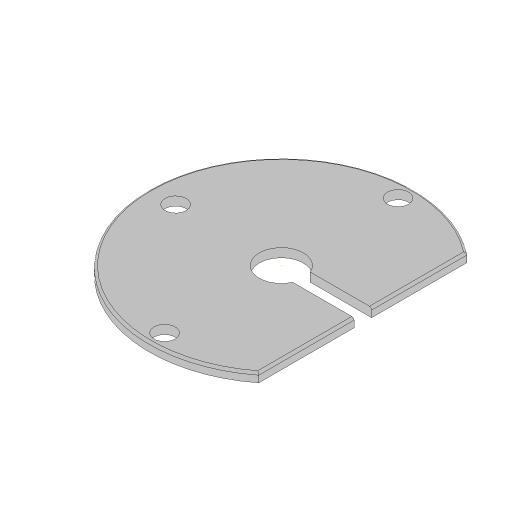
# Autodesk Inventor part: webcam_holder_center_part2
Saved by Autodesk Inventor 2023 (Build 270158000, 158)
## iProperties
Created: 2024-01-25
Part Number: webcam_holder_center_part2
Material: Generic
Document SubType Name: Modeling
Designer: qg3473
Density: 1 g/cm^3
Appearance: Default
Author: qg3473
Autodesk Inventor part; units mm, degrees
ref_plane "YZ Plane" through (0, 0, 0) normal (1, 0, 0) x (0, 1, 0)
ref_plane "XZ Plane" through (0, 0, 0) normal (0, 1, 0) x (-1, 0, 0)
ref_plane "XY Plane" through (0, 0, 0) normal (0, 0, 1) x (1, 0, 0)
sketch "Sketch1" plane through (0, 0, 0) normal (0, 1, 0) x (-1, 0, 0)
  arc A0 (-18.5, -23.6167) -> (-18.5, 23.6167) centre (0, 0) ccw
  line L0 (30, 0) -> (24, 0)
  circle A1 centre (24, 0) radius 2.4
  line L1 (0, 30) -> (0, 26.5)
  line L2 (0, -30) -> (0, -26.5)
  circle A2 centre (0, 26.5) radius 2.4
  circle A3 centre (0, -26.5) radius 2.4
  circle A4 centre (0, 0) radius 5
  line L3 (-30, 0) -> (-18.5, 0)
  line L4 (-18.5, 23.6167) -> (-18.5, -23.6167)
  dimension "d0" = 60
  dimension "d1" = 6
  dimension "d2" = 4.8
  dimension "d3" = 3.5
  dimension "d4" = 3.5
  dimension "d5" = 4.8
  dimension "d6" = 4.8
  dimension "d7" = 10
  dimension "d8" = 11.5
  constraints: 10 end point, 5 centre point, 5 coincident, 5 point on circle, 3 vertical, 2 horizontal
  measures "d0" diameter of A0
  measures "d1" distance of L0.start L0.end
  measures "d2" diameter of A1
  measures "d3" distance of L1.start L1.end
  measures "d4" distance of L2.start L2.end
  measures "d5" diameter of A2
  measures "d6" diameter of A3
  measures "d7" diameter of A4
  measures "d8" distance of L3.start L3.end
extrude "Extrusion1" add sketch "Sketch1" along normal blind 2
sketch "Sketch2" plane through (0, 2, 0) normal (0, 1, 0) x (1, 0, 0)
  point P0 (0, 0)
sketch "Sketch3" plane through (0, 2, 0) normal (0, 1, 0) x (1, 0, 0)
  point P0 (0, 0)
sketch "Sketch4" plane through (0, 0, 0) normal (0, -1, 0) x (1, 0, 0)
  line L0 (21.8231, -2) -> (3.4171, -2)
  line L1 (3.4171, -2) -> (3.4171, 2)
  line L2 (3.4171, 2) -> (21.8231, 2)
  line L3 (21.8231, 2) -> (21.8231, -2)
  line L4 (21.8231, -2) -> (3.4171, 2) construction
  line L5 (3.4171, -2) -> (21.8231, 2) construction
  point P0 (0, 0)
  point P1 (12.6201, 0)
  dimension "d17" = 4
  constraints: 12 end point, 2 midpoint, 2 parallel, 1 horizontal, 1 perpendicular
  measures "d17" distance of L0.end L1.end
extrude "Extrusion2" cut sketch "Sketch4" against normal blind 3
fillet "Fillet1" radius 0.5 3 edges at (-30, 2, 0) (18.5, 2, -12.8084) (18.5, 2, 12.8084)
body "Solid1"
